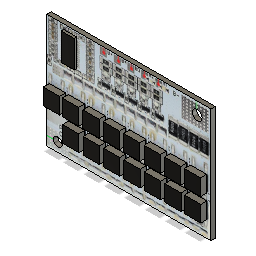
5S100ABMS v1 (Autodesk Fusion 360 design; units mm, degrees)
Autodesk Fusion 360 part; units mm, degrees
sketch "Sketch1" plane through (0, 0, 0) normal (0, 0, 1) x (1, 0, 0) in component "5S100ABMS"
  line L0 (-30.4, 21.15) -> (30.4, 21.15)
  line L1 (30.4, 21.15) -> (30.4, -21.15)
  line L2 (30.4, -21.15) -> (-30.4, -21.15)
  line L3 (-30.4, -21.15) -> (-30.4, 21.15)
  line L4 (-30.4, 21.15) -> (30.4, -21.15) construction
  line L5 (30.4, 21.15) -> (-30.4, -21.15) construction
  line L6 (30.4, 21.15) -> (27.1, 21.15) construction
  line L7 (27.1, 21.15) -> (27.1, 18.45) construction
  line L8 (27.1, 18.45) -> (30.4, 18.45) construction
  line L9 (30.4, 18.45) -> (30.4, 21.15) construction
  line L10 (-30.4, -19.35) -> (-27.9, -19.35) construction
  line L11 (-27.9, -19.35) -> (-27.9, -21.15) construction
  line L12 (-27.9, -21.15) -> (-30.4, -21.15) construction
  line L13 (-30.4, -21.15) -> (-30.4, -19.35) construction
  circle A0 centre (25.3, 16.65) radius 1.8
  circle A1 centre (-26.3, -17.75) radius 1.6
  line L14 (25.3, 16.65) -> (27.1, 16.65) construction
  line L15 (27.1, 16.65) -> (27.1, 18.45) construction
  line L16 (27.1, 18.45) -> (25.3, 18.45) construction
  line L17 (25.3, 18.45) -> (25.3, 16.65) construction
  line L18 (-26.3, -17.75) -> (-27.9, -17.75) construction
  line L19 (-27.9, -17.75) -> (-27.9, -19.35) construction
  line L20 (-27.9, -19.35) -> (-26.3, -19.35) construction
  line L21 (-26.3, -19.35) -> (-26.3, -17.75) construction
  dimension "Length" = 60.8
  dimension "Width" = 42.3
  dimension "d3" = 3.3
  dimension "d4" = 2.7
  dimension "d5" = 2.5
  dimension "d6" = 1.8
  dimension "d7" = 3.6
  dimension "d8" = 3.2
  constraint horizontal L0
  constraint perpendicular L0 L1
  constraint parallel L0 L2
  constraint parallel L1 L3
  constraint coincident L4 origin
  constraint coincident L5 origin
  constraint horizontal L6
  constraint vertical L7
  constraint horizontal L8
  constraint vertical L9
  constraint horizontal L10
  constraint vertical L11
  constraint horizontal L12
  constraint vertical L13
  constraint coincident L0.end L1.start
  constraint coincident L2.end L3.start
  constraint horizontal L14
  constraint vertical L15
  constraint horizontal L16
  constraint vertical L17
  constraint coincident A0.centre L14.start
  constraint tangent A0 L15
  constraint tangent A0 L16
  constraint coincident L7.end L8.start
  constraint horizontal L18
  constraint vertical L19
  constraint horizontal L20
  constraint vertical L21
  constraint coincident A1.centre L18.start
  constraint tangent A1 L20
  constraint tangent A1 L19
  constraint coincident L10.end L11.start
  measures "Length" distance of L1.end L2.end
  measures "Width" distance of L0.end L1.end
  measures "d3" distance of L0.end L6.end
  measures "d4" distance of L0.end L8.end
  measures "d5" distance of L10.start L10.end
  measures "d6" distance of L10.start L2.end
  measures "d7" diameter of A0
  measures "d8" diameter of A1
extrude "Extrude1" add sketch "Sketch1" along normal blind 1.6 in component "5S100ABMS"
sketch "Sketch2" plane through (0, 0, 1.6) normal (0, 0, 1) x (1, 0, 0) in component "5S100ABMS"
  circle A0 centre (-26.3, -17.75) radius 1.6
  circle A1 centre (25.3, 16.65) radius 1.8
  line L0 (-30.4, -21.15) -> (30.4, -21.15)
  line L1 (30.4, -21.15) -> (30.4, 21.15)
  line L2 (30.4, 21.15) -> (-30.4, 21.15)
  line L3 (-30.4, 21.15) -> (-30.4, -21.15)
  line L4 (-29.4367, -6.6251) -> (-29.4367, -0.6251)
  line L5 (-23.4367, -0.6251) -> (-23.4367, -6.6251)
  line L6 (-29.4367, -0.6251) -> (-23.4367, -0.6251)
  line L7 (-29.4367, -6.6251) -> (-23.4367, -0.6251) construction
  line L8 (-23.4367, -6.6251) -> (-29.4367, -6.6251)
  line L9 (-23.4367, -6.6251) -> (-29.4367, -0.6251) construction
  line L10 (-22.2878, -15.0909) -> (-22.2878, -9.0909)
  line L11 (-16.2878, -9.0909) -> (-16.2878, -15.0909)
  line L12 (-22.2878, -9.0909) -> (-16.2878, -9.0909)
  line L13 (-22.2878, -15.0909) -> (-16.2878, -9.0909) construction
  line L14 (-16.2878, -15.0909) -> (-22.2878, -15.0909)
  line L15 (-16.2878, -15.0909) -> (-22.2878, -9.0909) construction
  line L16 (-14.6686, -15.0909) -> (-14.6686, -9.0909)
  line L17 (-8.6686, -9.0909) -> (-8.6686, -15.0909)
  line L18 (-14.6686, -9.0909) -> (-8.6686, -9.0909)
  line L19 (-14.6686, -15.0909) -> (-8.6686, -9.0909) construction
  line L20 (-8.6686, -15.0909) -> (-14.6686, -15.0909)
  line L21 (-8.6686, -15.0909) -> (-14.6686, -9.0909) construction
  line L22 (-7.1435, -15.0909) -> (-7.1435, -9.0909)
  line L23 (-1.1435, -9.0909) -> (-1.1435, -15.0909)
  line L24 (-7.1435, -9.0909) -> (-1.1435, -9.0909)
  line L25 (-7.1435, -15.0909) -> (-1.1435, -9.0909) construction
  line L26 (-1.1435, -15.0909) -> (-7.1435, -15.0909)
  line L27 (-1.1435, -15.0909) -> (-7.1435, -9.0909) construction
  line L28 (0.3817, -15.0909) -> (0.3817, -9.0909)
  line L29 (6.3817, -9.0909) -> (6.3817, -15.0909)
  line L30 (0.3817, -9.0909) -> (6.3817, -9.0909)
  line L31 (0.3817, -15.0909) -> (6.3817, -9.0909) construction
  line L32 (6.3817, -15.0909) -> (0.3817, -15.0909)
  line L33 (6.3817, -15.0909) -> (0.3817, -9.0909) construction
  line L34 (7.9839, -15.0909) -> (7.9839, -9.0909)
  line L35 (13.9839, -9.0909) -> (13.9839, -15.0909)
  line L36 (7.9839, -9.0909) -> (13.9839, -9.0909)
  line L37 (7.9839, -15.0909) -> (13.9839, -9.0909) construction
  line L38 (13.9839, -15.0909) -> (7.9839, -15.0909)
  line L39 (13.9839, -15.0909) -> (7.9839, -9.0909) construction
  line L40 (15.5731, -15.0909) -> (15.5731, -9.0909)
  line L41 (21.5731, -9.0909) -> (21.5731, -15.0909)
  line L42 (15.5731, -9.0909) -> (21.5731, -9.0909)
  line L43 (15.5731, -15.0909) -> (21.5731, -9.0909) construction
  line L44 (21.5731, -15.0909) -> (15.5731, -15.0909)
  line L45 (21.5731, -15.0909) -> (15.5731, -9.0909) construction
  line L46 (22.9058, -15.0909) -> (22.9058, -9.0909)
  line L47 (28.9058, -9.0909) -> (28.9058, -15.0909)
  line L48 (22.9058, -9.0909) -> (28.9058, -9.0909)
  line L49 (22.9058, -15.0909) -> (28.9058, -9.0909) construction
  line L50 (28.9058, -15.0909) -> (22.9058, -15.0909)
  line L51 (28.9058, -15.0909) -> (22.9058, -9.0909) construction
  line L52 (-16.3819, -6.6251) -> (-22.3819, -6.6251)
  line L53 (-1.2375, -6.6251) -> (-7.2375, -0.6251) construction
  line L54 (0.2876, -6.6251) -> (0.2876, -0.6251)
  line L55 (-1.2375, -0.6251) -> (-1.2375, -6.6251)
  line L56 (7.9089, -6.6251) -> (7.9089, -0.6251)
  line L57 (13.9089, -6.6251) -> (7.9089, -0.6251) construction
  line L58 (-22.3819, -6.6251) -> (-16.3819, -0.6251) construction
  line L59 (-16.3819, -6.6251) -> (-22.3819, -0.6251) construction
  line L60 (28.8058, -6.6251) -> (22.8058, -6.6251)
  line L61 (6.2876, -0.6251) -> (6.2876, -6.6251)
  line L62 (-14.7627, -6.6251) -> (-14.7627, -0.6251)
  line L63 (15.479, -6.6251) -> (21.479, -0.6251) construction
  line L64 (-1.2375, -6.6251) -> (-7.2375, -6.6251)
  line L65 (-14.7627, -6.6251) -> (-8.7627, -0.6251) construction
  line L66 (22.8058, -6.6251) -> (22.8058, -0.6251)
  line L67 (-7.2375, -6.6251) -> (-7.2375, -0.6251)
  line L68 (7.9089, -0.6251) -> (13.9089, -0.6251)
  line L69 (22.8058, -6.6251) -> (28.8058, -0.6251) construction
  line L70 (21.479, -6.6251) -> (15.479, -0.6251) construction
  line L71 (28.8058, -0.6251) -> (28.8058, -6.6251)
  line L72 (0.2876, -0.6251) -> (6.2876, -0.6251)
  line L73 (-22.3819, -0.6251) -> (-16.3819, -0.6251)
  line L74 (13.9089, -0.6251) -> (13.9089, -6.6251)
  line L75 (-8.7627, -0.6251) -> (-8.7627, -6.6251)
  line L76 (-16.3819, -0.6251) -> (-16.3819, -6.6251)
  line L77 (22.8058, -0.6251) -> (28.8058, -0.6251)
  line L78 (21.479, -0.6251) -> (21.479, -6.6251)
  line L79 (15.479, -0.6251) -> (21.479, -0.6251)
  line L80 (-7.2375, -6.6251) -> (-1.2375, -0.6251) construction
  line L81 (-8.7627, -6.6251) -> (-14.7627, -6.6251)
  line L82 (28.8058, -6.6251) -> (22.8058, -0.6251) construction
  line L83 (-14.7627, -0.6251) -> (-8.7627, -0.6251)
  line L84 (-22.3819, -6.6251) -> (-22.3819, -0.6251)
  line L85 (7.9089, -6.6251) -> (13.9089, -0.6251) construction
  line L86 (0.2876, -6.6251) -> (6.2876, -0.6251) construction
  line L87 (-7.2375, -0.6251) -> (-1.2375, -0.6251)
  line L88 (13.9089, -6.6251) -> (7.9089, -6.6251)
  line L89 (-8.7627, -6.6251) -> (-14.7627, -0.6251) construction
  line L90 (21.479, -6.6251) -> (15.479, -6.6251)
  line L91 (6.2876, -6.6251) -> (0.2876, -6.6251)
  line L92 (6.2876, -6.6251) -> (0.2876, -0.6251) construction
  line L93 (15.479, -6.6251) -> (15.479, -0.6251)
  line L94 (-24.0917, 19.3813) -> (-19.3155, 19.3813)
  line L95 (-19.3155, 19.3813) -> (-19.3155, 9.2896)
  line L96 (-19.3155, 9.2896) -> (-24.0917, 9.2896)
  line L97 (-24.0917, 9.2896) -> (-24.0917, 19.3813)
  point P0 (-26.4367, -3.6251)
  point P1 (-19.3819, -3.6251)
  point P2 (-19.2878, -12.0909)
  point P3 (-11.6686, -12.0909)
  point P4 (-4.1435, -12.0909)
  point P5 (3.3817, -12.0909)
  point P6 (10.9839, -12.0909)
  point P7 (18.5731, -12.0909)
  point P8 (25.9058, -12.0909)
  point P9 (-19.3819, -3.6251)
  point P10 (10.9089, -3.6251)
  point P11 (-11.7627, -3.6251)
  point P12 (18.479, -3.6251)
  point P13 (3.2876, -3.6251)
  point P14 (-4.2375, -3.6251)
  point P15 (25.8058, -3.6251)
  dimension "d13" = 6
  dimension "d14" = 6
  dimension "d17" = 6
  dimension "d18" = 6
  dimension "d19" = 6
  dimension "d20" = 6
  dimension "d21" = 6
  dimension "d22" = 6
  dimension "d23" = 6
  dimension "d24" = 6
  dimension "d25" = 6
  dimension "d26" = 6
  dimension "d27" = 6
  dimension "d28" = 6
  dimension "d29" = 6
  dimension "d30" = 6
  dimension "d31" = 6
  dimension "d32" = 6
  dimension "d33" = 6
  dimension "d34" = 6
  dimension "d35" = 6
  dimension "d36" = 6
  dimension "d37" = 6
  dimension "d38" = 6
  dimension "d39" = 6
  dimension "d40" = 6
  dimension "d41" = 6
  dimension "d42" = 6
  dimension "d43" = 6
  dimension "d44" = 6
  dimension "d45" = 4.7762
  constraint horizontal L8
  constraint perpendicular L4 L8
  constraint parallel L6 L8
  constraint parallel L4 L5
  constraint coincident P0 L9
  constraint coincident P0 L7
  constraint horizontal L14
  constraint perpendicular L10 L14
  constraint parallel L12 L14
  constraint parallel L10 L11
  constraint coincident P2 L15
  constraint coincident P2 L13
  constraint horizontal L20
  constraint perpendicular L16 L20
  constraint parallel L18 L20
  constraint parallel L16 L17
  constraint coincident P3 L21
  constraint coincident P3 L19
  constraint horizontal L26
  constraint perpendicular L22 L26
  constraint parallel L24 L26
  constraint parallel L22 L23
  constraint coincident P4 L27
  constraint coincident P4 L25
  constraint horizontal L32
  constraint perpendicular L28 L32
  constraint parallel L30 L32
  constraint parallel L28 L29
  constraint coincident P5 L33
  constraint coincident P5 L31
  constraint horizontal L38
  constraint perpendicular L34 L38
  constraint parallel L36 L38
  constraint parallel L34 L35
  constraint coincident P6 L39
  constraint coincident P6 L37
  constraint horizontal L44
  constraint perpendicular L40 L44
  constraint parallel L42 L44
  constraint parallel L40 L41
  constraint coincident P7 L45
  constraint coincident P7 L43
  constraint horizontal L50
  constraint perpendicular L46 L50
  constraint parallel L48 L50
  constraint parallel L46 L47
  constraint coincident P8 L51
  constraint coincident P8 L49
  constraint collinear L12 L18
  constraint collinear L18 L24
  constraint collinear L24 L30
  constraint collinear L30 L36
  constraint collinear L36 L42
  constraint collinear L42 L48
  constraint horizontal L52
  constraint perpendicular L52 L84
  constraint parallel L52 L73
  constraint parallel L76 L84
  constraint coincident P9 L59
  constraint coincident P9 L58
  constraint horizontal L81
  constraint perpendicular L62 L81
  constraint parallel L81 L83
  constraint parallel L62 L75
  constraint coincident P11 L89
  constraint coincident P11 L65
  constraint horizontal L64
  constraint perpendicular L64 L67
  constraint parallel L64 L87
  constraint parallel L55 L67
  constraint coincident P14 L53
  constraint coincident P14 L80
  constraint horizontal L91
  constraint perpendicular L54 L91
  constraint parallel L72 L91
  constraint parallel L54 L61
  constraint coincident P13 L92
  constraint coincident P13 L86
  constraint horizontal L88
  constraint perpendicular L56 L88
  constraint parallel L68 L88
  constraint parallel L56 L74
  constraint coincident P10 L57
  constraint coincident P10 L85
  constraint horizontal L90
  constraint perpendicular L90 L93
  constraint parallel L79 L90
  constraint parallel L78 L93
  constraint coincident P12 L70
  constraint coincident P12 L63
  constraint horizontal L60
  constraint perpendicular L60 L66
  constraint parallel L60 L77
  constraint parallel L66 L71
  constraint coincident P15 L82
  constraint coincident P15 L69
  constraint collinear L73 L83
  constraint collinear L83 L87
  constraint collinear L72 L87
  constraint collinear L68 L72
  constraint collinear L68 L79
  constraint collinear L77 L79
  constraint coincident P9 P1
  constraint collinear L6 L73
  constraint horizontal L94
  constraint vertical L95
  constraint horizontal L96
  constraint vertical L97
  measures "d13" distance of L4.end L5.start
  measures "d14" distance of L4.end L4.start
  measures "d17" distance of L10.end L11.start
  measures "d18" distance of L10.end L10.start
  measures "d19" distance of L16.end L17.start
  measures "d20" distance of L16.end L16.start
  measures "d21" distance of L22.end L23.start
  measures "d22" distance of L22.end L22.start
  measures "d23" distance of L28.end L29.start
  measures "d24" distance of L28.end L28.start
  measures "d25" distance of L34.end L35.start
  measures "d26" distance of L34.end L34.start
  measures "d27" distance of L40.end L41.start
  measures "d28" distance of L40.end L40.start
  measures "d29" distance of L46.end L47.start
  measures "d30" distance of L46.end L46.start
  measures "d31" distance of L59.end L58.end
  measures "d32" distance of L52.end L59.end
  measures "d33" distance of L62.end L65.end
  measures "d34" distance of L62.end L62.start
  measures "d35" distance of L53.end L55.start
  measures "d36" distance of L53.end L64.end
  measures "d37" distance of L61.start L54.end
  measures "d38" distance of L54.start L54.end
  measures "d39" distance of L68.end L56.end
  measures "d40" distance of L56.end L56.start
  measures "d41" distance of L70.end L63.end
  measures "d42" distance of L63.start L70.end
  measures "d43" distance of L66.end L69.end
  measures "d44" distance of L66.end L60.end
  measures "d45" distance of L94.start L94.end
extrude "Extrude2" add sketch "Sketch2" along normal blind 0.94 contours L94 L95 L96 L97 in component "5S100ABMS"
extrude "Extrude3" add sketch "Sketch2" along normal blind 2.25 contours L4 L5 L6 L8 | L10 L11 L12 L14 | L16 L17 L18 L20 | L22 L23 L24 L26 | L28 L29 L30 L32 | L34 L35 L36 L38 | L40 L41 L42 L44 | L46 L47 L48 L50 | L52 L73 L76 L84 | L54 L61 L72 L91 | L55 L64 L67 L87 | L56 L68 L74 L88 | L60 L66 L71 L77 | L62 L75 L81 L83 | L78 L79 L90 L93 in component "5S100ABMS"
component "5S100ABMS" placed x (1, 0, 0) y (0, 1, 0) z (0, 0, 1) at (0, 0, 0)
equation "Thickness = 1.6 mm"
equation "d46 = 2.54 mm - Thickness"
equation "d48 = 3.85 mm - Thickness"
named bodies: "5S100ABMS"
